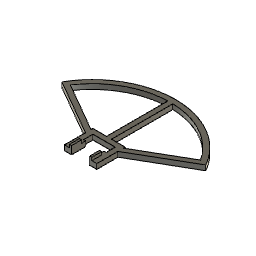
Prop_guard_clamp_new v1 (Autodesk Fusion 360 design; units mm, degrees)
Autodesk Fusion 360 part; units mm, degrees
sketch "Sketch1" plane through (0, 0, 0) normal (0, 0, 1) x (1, 0, 0)
  line L0 (-15.148, 8.7457) -> (-67.55, 39)
  arc A0 (67.55, 39) -> (-67.55, 39) centre (0, 0) ccw
  line L1 (-10.448, 11) -> (10.552, 11)
  line L2 (10.552, 11) -> (10.552, 2.4)
  line L3 (-10.448, 2.4) -> (-10.448, 11)
  line L4 (-10.448, -11.019) -> (-15.148, -11.019)
  line L5 (10.552, -11.019) -> (15.252, -11.019)
  line L6 (-15.148, 15.681) -> (-2.35, 15.681)
  line L7 (15.252, 8.8057) -> (67.55, 39)
  line L8 (15.252, 14.0679) -> (61.0783, 40.5257)
  line L9 (-15.148, 13.9229) -> (-61.119, 40.4642)
  line L10 (0, 73.3) -> (0.052, 73.3)
  line L11 (0.052, 15.681) -> (0, 15.681)
  line L12 (2.35, 50) -> (2.35, 15.681)
  line L13 (2.35, 50) -> (2.35, 73.2623)
  line L14 (-2.35, 44.2473) -> (-2.35, 15.681)
  line L15 (-2.35, 44.2473) -> (-2.35, 73.2623)
  line L16 (2.35, 15.681) -> (15.252, 15.681)
  arc A1 (61.0783, 40.5257) -> (2.35, 73.2623) centre (0, 0) ccw
  arc A2 (-2.35, 73.2623) -> (-61.119, 40.4642) centre (0, 0) ccw
  line L17 (-15.148, -11.019) -> (-15.148, 8.7457)
  line L18 (-15.148, 13.9229) -> (-15.148, 15.681)
  line L19 (15.252, -11.019) -> (15.252, 8.8057)
  line L20 (15.252, 14.0679) -> (15.252, 15.681)
  line L21 (-10.448, -11.019) -> (-8.448, -11.019)
  line L22 (10.552, -11.019) -> (8.552, -11.019)
  line L23 (-8.448, -11.019) -> (-8.448, 2.4)
  line L24 (-8.448, 2.4) -> (-10.448, 2.4)
  line L25 (8.552, -11.019) -> (8.552, 2.4)
  line L26 (8.552, 2.4) -> (10.552, 2.4)
  dimension "d11" = 26.7
  dimension "d15" = 2
  dimension "d16" = 2
  dimension "d17" = 13.419
  dimension "d18" = 13.419
  constraint horizontal L1
  constraint vertical L2
  constraint vertical L3
  constraint perpendicular L3 L4
  constraint perpendicular L2 L5
  constraint perpendicular L4 L17
  constraint perpendicular L5 L19
  constraint coincident L8.start L19
  constraint parallel L7 L8
  constraint coincident L9.start L17
  constraint parallel L0 L9
  constraint horizontal L10
  constraint horizontal L11
  constraint perpendicular L6 L12
  constraint perpendicular L6 L14
  constraint coincident L6 L11.start
  constraint perpendicular L12 L16
  constraint perpendicular L3 L21
  constraint perpendicular L2 L22
  constraint perpendicular L21 L23
  constraint perpendicular L3 L24
  constraint perpendicular L22 L25
  constraint perpendicular L2 L26
  measures "d11" distance of L5.end L16.end
  measures "d15" distance of L4.start L21.end
  measures "d16" distance of L5.start L22.end
  measures "d17" distance of L21.end L23.end
  measures "d18" distance of L22.end L25.end
extrude "Extrude1" add sketch "Sketch1" along normal blind 4.7
sketch "Sketch2" plane through (0, 0, 4.7) normal (0, 0, 1) x (-1, 0, 0)
  arc A0 (-61.0783, -40.5257) -> (-2.35, -73.2623) centre (0, 0) ccw
  line L0 (-61.0783, -40.5257) -> (-15.252, -14.0679)
  line L1 (-15.252, -14.0679) -> (-15.252, -15.681)
  line L2 (-15.252, -15.681) -> (-2.35, -15.681)
  line L3 (-2.35, -15.681) -> (-2.35, -73.2623)
  line L4 (2.35, -73.2623) -> (2.35, -15.681)
  line L5 (2.35, -15.681) -> (15.148, -15.681)
  line L6 (15.148, -15.681) -> (15.148, -13.9229)
  line L7 (15.148, -13.9229) -> (61.119, -40.4642)
  arc A1 (2.35, -73.2623) -> (61.119, -40.4642) centre (0, 0) ccw
  line L8 (-8.552, 11.019) -> (-15.252, 11.019)
  line L9 (-15.252, 11.019) -> (-15.252, -8.8057)
  line L10 (-15.252, -8.8057) -> (-67.55, -39)
  arc A2 (-67.55, -39) -> (67.55, -39) centre (0, 0) ccw
  line L11 (67.55, -39) -> (15.148, -8.7457)
  line L12 (15.148, -8.7457) -> (15.148, 11.019)
  line L13 (15.148, 11.019) -> (8.448, 11.019)
  line L14 (8.448, 11.019) -> (8.448, -2.4)
  line L15 (8.448, -2.4) -> (10.448, -2.4)
  line L16 (10.448, -2.4) -> (10.448, -11)
  line L17 (10.448, -11) -> (-10.552, -11)
  line L18 (-10.552, -11) -> (-10.552, -2.4)
  line L19 (-10.552, -2.4) -> (-8.552, -2.4)
  line L20 (-8.552, -2.4) -> (-8.552, 11.019)
  line L21 (8.448, 1.6) -> (10.448, 1.6)
  line L22 (10.448, 1.6) -> (10.448, 11.019)
  line L23 (-8.552, 1.6) -> (-10.552, 1.6)
  line L24 (-10.552, 1.6) -> (-10.552, 11.019)
  dimension "d21" = 9.419
  dimension "d22" = 9.419
  dimension "d23" = 2
  constraint coincident L13 L22.end
  constraint perpendicular L13 L22
  constraint coincident L8 L24.end
  constraint perpendicular L8 L24
  measures "d21" distance of L13.end L21.start
  measures "d22" distance of L8.start L23.start
  measures "d23" distance of L23.start L23.end
extrude "Extrude2" add sketch "Sketch2" along normal blind 2.8 contours L8 L20 L23 L24 | L13 L14 L21 L22
